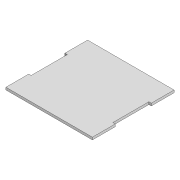
# Autodesk Inventor part: Gel base
Saved by Autodesk Inventor 2020 (Build 240168000, 168)
## iProperties
Created: 2022-04-26
Part Number: Gel base
Material: Generic
Document SubType Name: Modeling
Designer: ferrerx
Density: 1 g/cm^3
Appearance: Default
Author: ferrerx
Autodesk Inventor part; units mm, degrees
ref_plane "YZ Plane" through (0, 0, 0) normal (1, 0, 0) x (0, 1, 0)
ref_plane "XZ Plane" through (0, 0, 0) normal (0, 1, 0) x (-1, 0, 0)
ref_plane "XY Plane" through (0, 0, 0) normal (0, 0, 1) x (1, 0, 0)
sketch "Sketch1" plane through (0, 0, 0) normal (0, 1, 0) x (-1, 0, 0)
  line L0 (90, 85) -> (-90, 85)
  line L1 (-90, 85) -> (-90, -85)
  line L2 (-90, -85) -> (90, -85)
  line L3 (90, -85) -> (90, 85)
  line L4 (90, 85) -> (-90, -85) construction
  line L5 (-90, 85) -> (90, -85) construction
  point P0 (0, 0)
  dimension "d0" = 170
  dimension "d1" = 180
  constraints: 12 end point, 2 midpoint, 2 parallel, 1 horizontal, 1 perpendicular
  measures "d0" distance of L0.end L1.end
  measures "d1" distance of L1.end L2.end
extrude "Extrusion1" add sketch "Sketch1" along normal blind 5
sketch "Sketch2" plane through (0, 5, 0) normal (0, 1, 0) x (1, 0, 0)
  line L0 (85, 37.5) -> (95, 37.5)
  line L1 (95, 37.5) -> (95, -37.5)
  line L2 (95, -37.5) -> (85, -37.5)
  line L3 (85, -37.5) -> (85, 37.5)
  line L4 (90, -85) -> (90, 85) projected
  line L5 (85, 37.5) -> (95, -37.5) construction
  line L6 (95, 37.5) -> (85, -37.5) construction
  line L7 (0, 0) -> (0, 85) construction
  line L8 (90, 85) -> (-90, 85) projected
  line L9 (-85, 37.5) -> (-95, 37.5)
  line L10 (-95, 37.5) -> (-95, -37.5)
  line L11 (-95, -37.5) -> (-85, -37.5)
  line L12 (-85, -37.5) -> (-85, 37.5)
  line L13 (-90, -85) -> (-90, 85)
  line L14 (-85, 37.5) -> (-95, -37.5) construction
  line L15 (-95, 37.5) -> (-85, -37.5) construction
  point P0 (90, 0)
  point P1 (-90, 0)
  dimension "d4" = 75
  dimension "d5" = 5
  constraints: 28 end point, 6 midpoint, 6 symmetric about line, 2 parallel, 1 horizontal, 1 perpendicular
  measures "d4" distance of L0.end L1.end
  measures "d5" distance between parallel lines of L4 L3
extrude "Extrusion2" cut sketch "Sketch2" against normal blind 10
body "Solid1"
